# Autodesk Inventor part: Pushbutton
Saved by Autodesk Inventor 2013 (Build 170138000, 138)
## iProperties
Created: 2013-01-27
Part Number: Pushbutton
Material: Generic
Document SubType Name: Modeling
Designer: davidgitz
Density: 1 g/cm^3
Author: davidgitz
Autodesk Inventor part; units mm, degrees
ref_plane "YZ Plane" through (0, 0, 0) normal (1, 0, 0) x (0, 1, 0)
ref_plane "XZ Plane" through (0, 0, 0) normal (0, 1, 0) x (-1, 0, 0)
ref_plane "XY Plane" through (0, 0, 0) normal (0, 0, 1) x (1, 0, 0)
sketch "FSM2JH, Pushbutton_60" plane through (0, 0, 0) normal (0, 0, 1) x (1, 0, 0)
  line L0 (1.6256, 0.254) -> (4.3688, 0.254)
  arc A0 (4.3688, 0.254) -> (5.1308, 0.9906) centre (4.3815, 1.0033) ccw
  line L1 (5.1308, 0.9906) -> (5.1308, 3.5052)
  arc A1 (5.1308, 3.5052) -> (4.3688, 4.2418) centre (4.3815, 3.4925) ccw
  line L2 (4.3688, 4.2418) -> (1.6256, 4.2418)
  arc A2 (1.6256, 4.2418) -> (0.8636, 3.5052) centre (1.6129, 3.4925) ccw
  line L3 (0.8636, 3.5052) -> (0.8636, 0.9906)
  arc A3 (0.8636, 0.9906) -> (1.6256, 0.254) centre (1.6129, 1.0033) ccw
  constraints: 8 end point, 8 point on circle, 4 centre point
extrude "Extrusion1" add sketch "FSM2JH, Pushbutton_60" along normal blind 6.35
body "Solid1"
